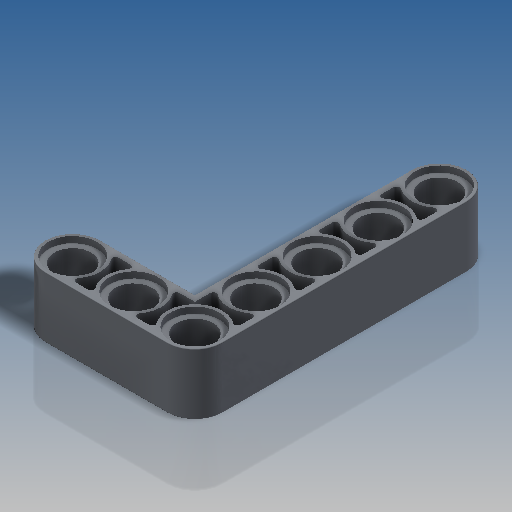
# Autodesk Inventor part: 32526-LtBluishGray
Saved by Autodesk Inventor 2019.4 (Build 234330000, 330)
## iProperties
Created: 2012-03-21
Part Number: 32526-LtBluishGray
Document SubType Name: Modeling
Designer: D. Kohfeld
Density: 1.06 g/cm^3
Material: ABS Plastic
Mass: 1.68001 g
Surface Area: 29.3688 cm^2
Volume: 1.58492 cm^3
Appearance: LtBluishGray
Author: D. Kohfeld
Autodesk Inventor part; units mm, degrees
ref_plane "YZ Plane" through (0, 0, 0) normal (1, 0, 0) x (0, 1, 0)
ref_plane "XZ Plane" through (0, 0, 0) normal (0, 1, 0) x (-1, 0, 0)
ref_plane "XY Plane" through (0, 0, 0) normal (0, 0, 1) x (1, 0, 0)
sketch "Sketch1" plane through (0, 0, 0) normal (0, 0, 1) x (1, 0, 0)
  line L0 (3.6, -20) -> (3.6, 12)
  line L1 (-3.6, 12) -> (-3.6, -16.4)
  arc A0 (3.6, 12) -> (-3.6, 12) centre (0, 12) ccw
  circle A1 centre (0, 4) radius 2.4
  circle A2 centre (0, 4) radius 3.2
  circle A3 centre (0, -4) radius 3.2
  circle A4 centre (0, -4) radius 2.4
  line L2 (0, -4) -> (0, 4) construction
  line L3 (-2.8, 1.7373) -> (-2.8, -1.7373)
  line L4 (2.8, 1.7373) -> (2.8, -1.7373)
  arc A5 (-2.8, 1.7373) -> (2.8, 1.7373) centre (0, 4) ccw
  arc A6 (2.8, -1.7373) -> (-2.8, -1.7373) centre (0, -4) ccw
  circle A7 centre (0, -20) radius 3.2
  circle A8 centre (0, -20) radius 2.4
  line L5 (-2.8, -14.2627) -> (-2.8, -17.7373)
  line L6 (2.8, -14.2627) -> (2.8, -17.7373)
  arc A9 (-2.8, -14.2627) -> (2.8, -14.2627) centre (0, -12) ccw
  arc A10 (2.8, -17.7373) -> (-2.8, -17.7373) centre (0, -20) ccw
  line L7 (0, 12) -> (0, 4) construction
  line L8 (2.8, 9.7373) -> (2.8, 6.2627)
  line L9 (-2.8, 9.7373) -> (-2.8, 6.2627)
  arc A11 (-2.8, 9.7373) -> (2.8, 9.7373) centre (0, 12) ccw
  arc A12 (2.8, 6.2627) -> (-2.8, 6.2627) centre (0, 4) ccw
  line L10 (-3.6, -16.4) -> (-16, -16.4)
  arc A13 (-16, -16.4) -> (-16, -23.6) centre (-16, -20) ccw
  line L11 (-16, -23.6) -> (0, -23.6)
  arc A14 (0, -23.6) -> (3.6, -20) centre (0, -20) ccw
  circle A15 centre (-16, -20) radius 3.2
  circle A16 centre (-16, -20) radius 2.4
  line L12 (-5.7373, -17.2) -> (-2.2627, -17.2)
  line L13 (-5.7373, -22.8) -> (-2.2627, -22.8)
  arc A17 (-2.2627, -17.2) -> (-2.2627, -22.8) centre (0, -20) ccw
  circle A18 centre (0, 12) radius 3.2
  circle A19 centre (0, 12) radius 2.4
  line L14 (-2.8, -6.2627) -> (-2.8, -9.7373)
  line L15 (2.8, -9.7373) -> (2.8, -6.2627)
  arc A20 (-2.8, -6.2627) -> (2.8, -6.2627) centre (0, -4) ccw
  arc A21 (2.8, -9.7373) -> (-2.8, -9.7373) centre (0, -12) ccw
  circle A22 centre (0, -12) radius 3.2
  circle A23 centre (0, -12) radius 2.4
  line L16 (0, -12) -> (0, -4) construction
  line L17 (0, -12) -> (0, -20) construction
  circle A24 centre (-8, -20) radius 3.2
  circle A25 centre (-8, -20) radius 2.4
  arc A26 (-5.7373, -22.8) -> (-5.7373, -17.2) centre (-8, -20) ccw
  line L18 (-10.2627, -17.2) -> (-13.7373, -17.2)
  line L19 (-13.7373, -22.8) -> (-10.2627, -22.8)
  arc A27 (-10.2627, -17.2) -> (-10.2627, -22.8) centre (-8, -20) ccw
  arc A28 (-13.7373, -22.8) -> (-13.7373, -17.2) centre (-16, -20) ccw
  line L20 (0, -20) -> (-8, -20) construction
  line L21 (-8, -20) -> (-16, -20) construction
  point P0 (0, 0)
  point P1 (0, 0)
  dimension "d8" = 4.8
  dimension "d9" = 6.4
  dimension "d32" = 7.2
  dimension "d34" = 8
  dimension "d36" = 0.8
  dimension "d49" = 0.8
  constraints: 44 end point, 30 point on circle, 29 centre point, 26 equal radius, 18 coincident, 13 equal length, 11 parallel, 6 tangent, 5 concentric, 4 vertical, 3 perpendicular, 3 vertical alignment, 2 collinear, 2 horizontal alignment, 1 midpoint
  measures "d8" diameter of A1
  measures "d9" diameter of A2
  measures "d32" diameter of A0
  measures "d34" distance of L2.start L2.end
  measures "d36" distance between parallel lines of L1 L3
  measures "d49" distance between parallel lines of L10 L12
extrude "Extrusion1" add sketch "Sketch1" along normal mid plane 8 contours A14 L11 A13 L10 L1 A0 L0 | A2 | A3 | A5 L4 A6 L3 | A7 | A9 L6 A10 L12 L5 | L12 A10 L5 | L5 A17 L13 A26 L12 | L8 A12 L9 A11 | A15 | A18 | A20 L15 A21 L14 | A22 | A24 | A27 L19 A28 L18
sketch "Sketch6" plane through (0, 0, 4) normal (0, 0, 1) x (1, 0, 0)
  circle A0 centre (0, -4) radius 3.2 projected
  circle A1 centre (0, 4) radius 3.2 projected
  arc A2 (2.8, -1.7373) -> (-2.8, -1.7373) centre (0, -4) ccw projected
  line L0 (-2.8, 1.7373) -> (-2.8, -1.7373) projected
  arc A3 (-2.8, 1.7373) -> (2.8, 1.7373) centre (0, 4) ccw projected
  line L1 (2.8, 1.7373) -> (2.8, -1.7373) projected
  line L2 (-2.8, -14.2627) -> (-2.8, -17.7373) projected
  arc A4 (-2.8, -14.2627) -> (2.8, -14.2627) centre (0, -12) ccw projected
  arc A5 (2.8, -17.7373) -> (-2.8, -17.7373) centre (0, -20) ccw projected
  line L3 (2.8, -14.2627) -> (2.8, -17.7373) projected
  circle A6 centre (0, -20) radius 3.2 projected
  circle A7 centre (0, -20) radius 2.4 projected
  line L4 (2.8, 9.7373) -> (2.8, 6.2627) projected
  arc A8 (-2.8, 9.7373) -> (2.8, 9.7373) centre (0, 12) ccw projected
  arc A9 (2.8, 6.2627) -> (-2.8, 6.2627) centre (0, 4) ccw projected
  line L5 (-2.8, 9.7373) -> (-2.8, 6.2627) projected
  line L6 (-5.7373, -17.2) -> (-2.2627, -17.2) projected
  arc A10 (-2.2627, -17.2) -> (-2.2627, -22.8) centre (0, -20) ccw projected
  line L7 (-5.7373, -22.8) -> (-2.2627, -22.8) projected
  circle A11 centre (-16, -20) radius 3.2 projected
  arc A12 (-5.7373, -22.8) -> (-5.7373, -17.2) centre (-8, -20) ccw projected
  circle A13 centre (-8, -20) radius 3.2 projected
  arc A14 (-10.2627, -17.2) -> (-10.2627, -22.8) centre (-8, -20) ccw projected
  line L8 (-13.7373, -22.8) -> (-10.2627, -22.8) projected
  arc A15 (-13.7373, -22.8) -> (-13.7373, -17.2) centre (-16, -20) ccw projected
  line L9 (-10.2627, -17.2) -> (-13.7373, -17.2) projected
  circle A16 centre (0, -12) radius 3.2 projected
  line L10 (2.8, -9.7373) -> (2.8, -6.2627) projected
  arc A17 (-2.8, -6.2627) -> (2.8, -6.2627) centre (0, -4) ccw projected
  line L11 (-2.8, -6.2627) -> (-2.8, -9.7373) projected
  arc A18 (2.8, -9.7373) -> (-2.8, -9.7373) centre (0, -12) ccw projected
  circle A19 centre (0, 12) radius 3.2 projected
extrude "Extrusion7" cut sketch "Sketch6" against normal blind 0.8 contours A0 | A1 | A6 | A7 | A11 | A13 | A16 | A19
extrude "Extrusion8" cut sketch "Sketch6" against normal blind 3.1 contours A2 L0 A3 L1 | A4 L3 A5 L6 L2 | L6 A5 L2 | L2 A10 L7 A12 L6 | L4 A9 L5 A8 | A14 L8 A15 L9 | A18 L11 A17 L10
mirror "Mirror1" about plane through (0, 0, 0) normal (0, 0, 1) of "Extrusion7", "Extrusion8"
fillet "Fillet1" radius 0.4 44 edges at (-2.8, -1.7373, 2.45) (-2.8, 1.7373, 2.45) (2.8, -1.7373, 2.45) (2.8, 1.7373, 2.45) (2.8, 1.7373, -2.45) (2.8, -1.7373, -2.45) (-2.8, -1.7373, -2.45) (-2.8, 1.7373, -2.45) (-2.8, -14.2627, 2.45) (2.8, -17.7373, 2.45) (2.8, -14.2627, 2.45) (2.8, -14.2627, -2.45) (2.8, -17.7373, -2.45) (-2.8, -14.2627, -2.45) (-5.7373, -17.2, 2.45) (-5.7373, -22.8, 2.45) (-2.2627, -22.8, 2.45) (-5.7373, -22.8, -2.45) (-2.2627, -22.8, -2.45) (-5.7373, -17.2, -2.45) (-2.8, 9.7373, 2.45) (-2.8, 6.2627, 2.45) (2.8, 6.2627, 2.45) (2.8, 9.7373, 2.45) (2.8, 6.2627, -2.45) (2.8, 9.7373, -2.45) (-2.8, 6.2627, -2.45) (-2.8, 9.7373, -2.45) (2.8, -6.2627, 2.45) (2.8, -6.2627, -2.45) (2.8, -9.7373, 2.45) (2.8, -9.7373, -2.45) (-2.8, -9.7373, 2.45) (-2.8, -6.2627, 2.45) (-2.8, -9.7373, -2.45) (-2.8, -6.2627, -2.45) (-10.2627, -22.8, 2.45) (-10.2627, -22.8, -2.45) (-13.7373, -22.8, 2.45) (-13.7373, -22.8, -2.45) (-13.7373, -17.2, 2.45) (-10.2627, -17.2, 2.45) (-13.7373, -17.2, -2.45) (-10.2627, -17.2, -2.45)
fillet "Fillet1" radius 0.1 6 edges at (-3.6, -2.2, 4) (0, 15.6, 4) (3.6, -4, 4) (0, 15.6, -4) (-3.6, -2.2, -4) (3.6, -4, -4)
body "Solid1"
